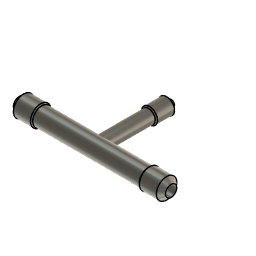
Connecteur essence en T - Grand (Autodesk Fusion 360 design; units mm, degrees)
Autodesk Fusion 360 part; units mm, degrees
sketch "Esquisse1" plane through (0, 0, 0) normal (1, 0, 0) x (0, 1, 0)
  circle A0 centre (0, 0) radius 2.5
  circle A1 centre (0, 0) radius 4
  dimension "d1" = 5
  dimension "d2" = 8
  constraint coincident A0.centre A1.centre
  constraint concentric A0 A1
  measures "d1" diameter of A0
  measures "d2" diameter of A1
extrude "Extrusion1" add sketch "Esquisse1" along normal blind 67 makes body 1
sketch "Esquisse2" plane through (0, 0, 0) normal (0, 1, 0) x (1, 0, 0)
  line L0 (0, -15) -> (0, 15) construction
  line L1 (67, -15) -> (67, 15) construction
  line L2 (33.5, -17) -> (33.5, 15) construction
  circle A0 centre (33.5, 0.0356) radius 1.5
  circle A1 centre (33.5, 0.0356) radius 3
  line L3 (36.4997, -0.0089) -> (30.5003, -0.0089) construction
  dimension "d5" = 67
  dimension "d7" = 33.5
  dimension "d8" = 33.5
  dimension "d9" = 3
  dimension "d10" = 6
  constraint vertical L0
  constraint vertical L1
  constraint vertical L2
  constraint coincident L2 A0.centre
  constraint concentric A0 A1
  constraint coincident A1 L3.start
  constraint coincident A1 L3.end
  constraint horizontal L3
  measures "d5" distance of L0.start L1.start
  measures "d7" distance of L1 L2
  measures "d8" distance of L0 L2
  measures "d9" diameter of A0
  measures "d10" diameter of A1
extrude "Extrusion2" add sketch "Esquisse2" along normal blind 33.5 separate body makes body 2
extrude "Extrusion3" cut sketch "Esquisse2" along normal blind 3 and the other way blind 2 contours A0 bodies 1
extrude "Extrusion4" cut sketch "Esquisse2" along normal blind 5 contours A0 bodies 1
extrude "Extrusion5" cut sketch "Esquisse1" along normal blind 67 contours A0 bodies 2
sketch "Esquisse3" plane through (0, 0, 0) normal (0, 0, 1) x (1, 0, 0)
  line L0 (5.0048, 5.9577) -> (5.0048, -6.0423) construction
  line L1 (0, 6) -> (0, -6) construction
  line L2 (67.0048, 5.9577) -> (67.0048, -6.0423) construction
  line L3 (62, 6) -> (62, -6) construction
  dimension "d22" = 5.0048
  dimension "d23" = 5.0048
  constraint vertical L0
  constraint parallel L0 L1
  constraint vertical L2
  constraint parallel L2 L3
  measures "d22" horizontal distance of L0.start L1.start
  measures "d23" horizontal distance of L3.start L2.start
sketch "Esquisse4" plane through (0, 0, 0) normal (1, 0, 0) x (0, 1, 0)
  circle A0 centre (0, 0) radius 4.5
  circle A1 centre (0, 0) radius 4
  dimension "d24" = 9
  dimension "d25" = 8
  constraint coincident A0.centre A1.centre
  constraint concentric A0 A1
  measures "d24" diameter of A0
  measures "d25" diameter of A1
extrude "Extrusion6" add sketch "Esquisse4" along normal blind 10 bodies 1
chamfer "Chanfrein1" distance 0.5 angle 45 1 edges at (10, -4.1955, -1.6273) on bodies 1
chamfer "Chanfrein2" distance 2 angle 45 1 edges at (0, -4.1955, -1.6273) on bodies 1
move_body "Déplacer1" bodies 1 2 to x (1, 0, 0) y (0, 1, 0) z (0, 0, 1) at (-67, 0, 0)
extrude "Extrusion7" add sketch "Esquisse4" against normal blind 10 bodies 1
chamfer "Chanfrein3" distance 0.5 angle 45 1 edges at (-10, -4.1955, 1.6273) on bodies 1
chamfer "Chanfrein4" distance 2 angle 45 1 edges at (0, -4.1955, -1.6273) on bodies 1
delete_face "DeleteFace1" 1 faces at (-33.4691, -1.9862, -1.5353) on bodies 1
sketch "Esquisse5" plane through (0, 33.5, 0) normal (0, 1, 0) x (-1, 0, 0)
  circle A0 centre (33.5, -0.0356) radius 1.5
  circle A1 centre (33.5, -0.0356) radius 3
  circle A2 centre (33.5, -0.0356) radius 1.5
  circle A3 centre (33.5, -0.0356) radius 3.5
  dimension "d35" = 7
  constraint concentric A0 A2
  constraint concentric A2 A3
  measures "d35" diameter of A3
extrude "Extrusion8" add sketch "Esquisse5" against normal blind 10 contours A3 bodies 2
chamfer "Chanfrein5" distance 2 angle 45 1 edges at (-30.2369, 33.5, -1.3012) on bodies 2
chamfer "Chanfrein6" distance 0.5 angle 45 1 edges at (-30.2369, 23.5, 1.2301) on bodies 2
sketch "Esquisse6" plane through (0, 0, 0) normal (1, 0, 0) x (0, 1, 0)
  line L0 (37, 0) -> (-4, 0)
  line L1 (-4, 0) -> (33.4768, 0)
  constraint horizontal L0
  constraint parallel L0 L1
move_body "Déplacer2" bodies 1 2 to x (1, 0, 0) y (0, 1, 0) z (0, 0, 1) at (33.5, 0, 0)
sketch "Esquisse7" plane through (0, 0, 0) normal (1, 0, 0) x (0, 1, 0)
  circle A0 centre (0, 0) radius 4.5
  circle A1 centre (0, 0) radius 4
  dimension "d40" = 9
  dimension "d41" = 8
  constraint coincident A0.centre A1.centre
  constraint concentric A0 A1
  measures "d40" diameter of A0
  measures "d41" diameter of A1
ref_plane "Plan de construction1" through (7, 0, 0) normal (1, 0, 0) x (0, 1, 0)
